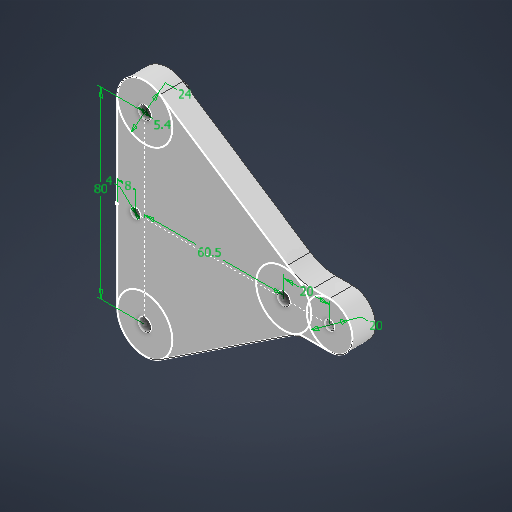
# Autodesk Inventor part: y axis something back
Saved by Autodesk Inventor 2025.1 (Build 291241000, 241)
## iProperties
Created: 2025-02-02
Part Number: y axis something back
Material: Generic
Document SubType Name: Modeling
Designer: jerem
Density: 1 g/cm^3
Appearance: Default
Author: jerem
Autodesk Inventor part; units mm, degrees
ref_plane "YZ Plane" through (0, 0, 0) normal (1, 0, 0) x (0, 1, 0)
ref_plane "XZ Plane" through (0, 0, 0) normal (0, 1, 0) x (-1, 0, 0)
ref_plane "XY Plane" through (0, 0, 0) normal (0, 0, 1) x (1, 0, 0)
sketch "Sketch1" plane through (0, 0, 0) normal (0, 0, 1) x (1, 0, 0)
  line L0 (0, 0) -> (30.25, 0) construction
  line L1 (0, 0) -> (-30.25, 0) construction
  line L2 (-30.25, 0) -> (-30.25, 40) construction
  line L3 (-30.25, 0) -> (-30.25, -40) construction
  circle A0 centre (-30.25, 40) radius 2.7
  circle A1 centre (-30.25, -40) radius 2.7
  circle A2 centre (30.25, 0) radius 2.7
  circle A3 centre (-30.25, 40) radius 12
  circle A4 centre (-30.25, -40) radius 12
  circle A5 centre (30.25, 0) radius 12
  line L4 (36.8682, -10.01) -> (-23.6318, -50.01)
  line L5 (-42.25, 40) -> (-42.25, -40)
  circle A6 centre (-34.25, 0) radius 2
  line L6 (-30.25, 0) -> (-34.25, 0) construction
  line L7 (-23.6318, 50.01) -> (36.8682, 10.01)
  line L8 (30.25, 0) -> (50.25, 0) construction
  circle A7 centre (50.25, 0) radius 10
  circle A8 centre (50.25, 0) radius 2
  line L9 (50.2575, 10) -> (36.8682, 10.01)
  line L10 (50.2575, -10) -> (36.8682, -10.01)
  point P0 (-42.25, 0)
  point P1 (41.35, -4.5596)
  point P2 (41.35, 4.5596)
  dimension "d0" = 60.5
  dimension "d1" = 5.4
  dimension "d2" = 80
  dimension "d3" = 24
  dimension "d55" = 4
  dimension "d56" = 8
  dimension "d57" = 20
  dimension "d58" = 20
  constraints: 22 end point, 9 centre point, 8 coincident, 8 point on circle, 7 tangent, 5 equal radius, 4 horizontal, 2 collinear, 2 vertical, 1 midpoint, 1 perpendicular
  measures "d0" distance of L0.end L1.end
  measures "d1" diameter of A0
  measures "d2" distance of L3.end L2.end
  measures "d3" diameter of A3
  measures "d55" diameter of A6
  measures "d56" distance of point (-42.25, 0) L6.end
  measures "d57" distance of L8.start L8.end
  measures "d58" diameter of A7
extrude "Extrusion1" add sketch "Sketch1" against normal blind 10
sketch "Sketch4" plane through (0, 0, -10) normal (0, 0, -1) x (1, 0, 0)
  arc A0 (-23.6318, 50.01) -> (-42.25, 40) centre (-30.25, 40) ccw projected
  arc A1 (-42.25, -40) -> (-23.6318, -50.01) centre (-30.25, -40) ccw projected
  circle A2 centre (-30.25, -40) radius 2.7 projected
  circle A3 centre (-30.25, -40) radius 4
  circle A4 centre (30.25, 0) radius 4
  circle A5 centre (-30.25, 40) radius 4
  line L0 (-42.25, 40) -> (-42.25, -40) projected
  line L1 (-23.6318, -50.01) -> (36.8682, -10.01) projected
  line L2 (36.8682, 10.01) -> (-23.6318, 50.01) projected
  arc A6 (50.2575, -10) -> (50.2575, 10) centre (50.25, 0) ccw projected
  line L3 (36.8682, -10.01) -> (50.2575, -10) projected
  line L4 (50.2575, 10) -> (36.8682, 10.01) projected
  point P0 (0, 0)
  dimension "d26" = 8
  constraints: 3 centre point, 2 equal radius, 1 coincident
  measures "d26" diameter of A3
extrude "Extrusion4" add sketch "Sketch4" along normal blind 6.45 contours A3 | A4 | A5
chamfer "Chamfer2" distance 6 angle 45 3 edges at (26.25, 0, -10) (-34.25, -40, -10) (-34.25, 40, -10)
fillet "Fillet1" radius 20 2 edges at (36.8682, 10.01, -5) (36.8682, -10.01, -5)
equation "\"b\" = 2"
body "Solid1"
